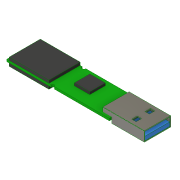
# Autodesk Inventor part: USB stick
Saved by Autodesk Inventor 2017 (Build 210142000, 142)
## iProperties
Part Number: USB stick
Material: Generisch
Document SubType Name: Modeling
Designer: ExCISS
Density: 1 g/cm^3
Appearance: Dunkelgrün
Author: ExCISS
Autodesk Inventor part; units mm, degrees
ref_plane "YZ Plane" through (0, 0, 0) normal (1, 0, 0) x (0, 1, 0)
ref_plane "XZ Plane" through (0, 0, 0) normal (0, 1, 0) x (-1, 0, 0)
ref_plane "XY Plane" through (0, 0, 0) normal (0, 0, 1) x (1, 0, 0)
sketch "Skizze1" plane through (0, 0, 0) normal (0, 0, 1) x (1, 0, 0)
  line L0 (-23.15, 7.05) -> (23.15, 7.05)
  line L1 (23.15, 7.05) -> (23.15, -7.05)
  line L2 (23.15, -7.05) -> (-23.15, -7.05)
  line L3 (-23.15, -7.05) -> (-23.15, 7.05)
  line L4 (-23.15, 7.05) -> (23.15, -7.05) construction
  point P0 (0, 0)
  point P1 (0, 0)
  dimension "d0" = 46.3
  dimension "d1" = 14.1
  constraints: 10 end point, 2 parallel, 1 coincident, 1 horizontal, 1 midpoint, 1 perpendicular
  measures "d0" distance of L1.end L2.end
  measures "d1" distance of L0.end L1.end
extrude "Extrusion1" add sketch "Skizze1" along normal blind 1
sketch "Skizze3" plane through (0, 0, 0) normal (0, 0, 1) x (1, 0, 0)
  line L0 (37.85, 6) -> (19.15, 6)
  line L1 (19.15, 6) -> (19.15, -6)
  line L2 (19.15, -6) -> (37.85, -6)
  line L3 (37.85, -6) -> (37.85, 6)
  line L4 (23.15, -7.05) -> (23.15, 7.05) projected
  line L5 (23.15, 0) -> (19.15, 0) construction
  point P0 (0, 0)
  dimension "d8" = 18.7
  dimension "d9" = 12
  constraints: 10 end point, 2 horizontal, 2 midpoint, 2 parallel, 1 perpendicular
  measures "d8" distance of L2.end L1.end
  measures "d9" distance of L1.end L0.end
extrude "Extrusion2" add sketch "Skizze3" along normal blind 2.9 separate body
sketch "Skizze4" plane through (0, 0, 0) normal (0, 0, -1) x (-1, 0, 0)
  line L0 (-19.15, -6) -> (-37.85, -6) projected
  line L1 (-23.15, -7.05) -> (-23.15, 7.05) projected
  line L2 (-37.85, -6) -> (-23.15, -6)
  line L3 (-23.15, -6) -> (-23.15, 6)
  line L4 (-23.15, 6) -> (-37.85, 6)
  line L5 (-37.85, 6) -> (-37.85, -6)
  point P0 (0, 0)
  dimension "d16" = 12
  constraints: 8 end point, 2 parallel, 1 horizontal, 1 perpendicular, 1 point on line
  measures "d16" distance of L3.end L2.end
extrude "Extrusion3" add sketch "Skizze4" along normal blind 1.6 bodies 2
sketch "Skizze5" plane through (0, 0, 1) normal (0, 0, 1) x (1, 0, 0)
  line L0 (-23.15, 7.05) -> (-23.15, -7.05) construction
  line L1 (23.15, 7.05) -> (-23.15, 7.05) construction
  line L2 (-22.15, 7.05) -> (-4.15, 7.05)
  line L3 (-4.15, 7.05) -> (-4.15, -7.05)
  line L4 (-4.15, -7.05) -> (-22.15, -7.05)
  line L5 (-22.15, -7.05) -> (-22.15, 7.05)
  point P0 (0, 0)
  dimension "d20" = 18
  dimension "d21" = 14.1
  constraints: 8 end point, 2 parallel, 1 horizontal, 1 perpendicular, 1 point on line
  measures "d20" distance of L3.end L4.end
  measures "d21" distance of L2.end L3.end
extrude "Extrusion4" add sketch "Skizze5" along normal blind 1.3 bodies 1
sketch "Skizze6" plane through (0, 0, 0) normal (0, 0, -1) x (-1, 0, 0)
  line L0 (23.15, 7.05) -> (23.15, -7.05) construction
  line L1 (23.15, 0) -> (22.15, 0) construction
  line L2 (22.15, 7.05) -> (22.15, -7.05) projected
  line L3 (22.15, -7.05) -> (4.15, -7.05)
  line L4 (4.15, -7.05) -> (4.15, 7.05)
  line L5 (4.15, 7.05) -> (22.15, 7.05)
  line L6 (22.15, 7.05) -> (22.15, -7.05)
  point P0 (0, 0)
  dimension "d24" = 1
  dimension "d25" = 18
  dimension "d26" = 14.1
  constraints: 10 end point, 2 horizontal, 2 parallel, 1 midpoint, 1 perpendicular
  measures "d24" distance of L1.start L1.end
  measures "d25" distance of L4.end L5.end
  measures "d26" distance of L3.end L4.end
extrude "Extrusion5" add sketch "Skizze6" along normal blind 1.3 bodies 1
sketch "Skizze8" plane through (37.85, -6, 2.9) normal (1, 0, 0) x (0, 0, -1)
  line L0 (4.5, 12) -> (4.5, 0) projected
  line L1 (0, 0) -> (0, 12) projected
  line L2 (0.35, 0.35) -> (2.35, 0.35)
  line L3 (2.35, 0.35) -> (2.35, 11.65)
  line L4 (2.35, 11.65) -> (0.35, 11.65)
  line L5 (0.35, 11.65) -> (0.35, 0.35)
  line L6 (0, 12) -> (0, 0) construction
  line L7 (0, 6) -> (0.35, 6) construction
  dimension "d42" = 2
  dimension "d43" = 11.3
  dimension "d44" = 0.35
  constraints: 10 end point, 2 horizontal, 2 midpoint, 2 parallel, 1 perpendicular
  measures "d42" distance of L4.end L3.end
  measures "d43" distance of L3.end L2.end
  measures "d44" distance of L7.end L7.start
extrude "Extrusion6" cut sketch "Skizze8" against normal blind 9 bodies 2
sketch "Skizze9" plane through (37.85, -6, 2.9) normal (1, 0, 0) x (0, 0, -1)
  line L0 (0, 0) -> (0, 12) projected
  line L1 (4.5, 12) -> (4.5, 0) projected
  line L2 (2.35, 11.65) -> (2.35, 0.35) projected
  line L3 (2.35, 0.35) -> (4.15, 0.35)
  line L4 (4.15, 0.35) -> (4.15, 11.65)
  line L5 (4.15, 11.65) -> (2.35, 11.65)
  line L6 (2.35, 11.65) -> (2.35, 0.35)
  point P0 (2.9, 6)
  constraints: 8 end point, 2 parallel, 1 horizontal, 1 perpendicular
extrude "Extrusion7" cut sketch "Skizze9" against normal blind 0.1 bodies 2
sketch "Skizze15" plane through (0, 0, 1) normal (0, 0, 1) x (1, 0, 0)
  line L0 (-4.1196, -7.0919) -> (-2.4201, -7.05) construction
  line L1 (-4.15, -7.05) -> (23.15, -7.05) construction
  circle A0 centre (-2.4201, -7.05) radius 0.7
  point P0 (0, 0)
  dimension "d81" = 1.7
  dimension "d82" = 1.4
  constraints: 2 end point, 1 centre point, 1 coincident, 1 point on line
  measures "d81" distance of L0.start L0.end
  measures "d82" diameter of A0
extrude "Extrusion8" cut sketch "Skizze15" against normal blind 1 bodies 1
sketch "Skizze17" plane through (0, 0, 1) normal (0, 0, 1) x (1, 0, 0)
  line L0 (-4.15, 7.05) -> (-22.15, 7.05) projected
  line L1 (-4.15, 7.05) -> (-2.45, 7.05)
  line L2 (23.15, 7.05) -> (-4.15, 7.05) projected
  circle A0 centre (-2.45, 7.05) radius 0.85
  point P0 (0, 0)
  dimension "d87" = 1.7
  dimension "d88" = 1.7
  constraints: 2 end point, 1 centre point, 1 coincident, 1 point on line
  measures "d87" distance of L0.start L1.end
  measures "d88" diameter of A0
extrude "Extrusion9" cut sketch "Skizze17" against normal blind 1 bodies 1
sketch "Skizze19" plane through (0, 0, 2.9) normal (0, 0, 1) x (1, 0, 0)
  line L0 (37.85, -6) -> (37.85, 6) projected
  line L1 (32.45, -4.25) -> (30.45, -4.25)
  line L2 (30.45, -4.25) -> (30.45, -1.75)
  line L3 (30.45, -1.75) -> (32.45, -1.75)
  line L4 (32.45, -1.75) -> (32.45, -4.25)
  point P0 (0, 0)
  point P1 (32.45, 4.25)
  dimension "d101" = 2
  dimension "d102" = 2.5
  constraints: 8 end point, 2 parallel, 1 horizontal, 1 perpendicular
  measures "d101" distance of L2.end L3.end
  measures "d102" distance of L1.end L2.end
extrude "Extrusion10" cut sketch "Skizze19" against normal up to next bodies 2
sketch "Skizze20" plane through (0, 0, 2.9) normal (0, 0, 1) x (1, 0, 0)
  line L0 (37.85, 5.65) -> (37.85, -5.65) projected
  line L1 (37.85, 0) -> (32.45, 0)
  line L2 (32.45, 0) -> (32.45, 4.25)
  line L3 (32.45, 4.25) -> (30.45, 4.25)
  line L4 (30.45, 4.25) -> (30.45, 1.75)
  line L5 (30.45, 1.75) -> (32.45, 1.75)
  line L6 (32.45, 1.75) -> (32.45, 4.25)
  point P0 (0, 0)
  dimension "d107" = 5.4
  dimension "d108" = 4.25
  dimension "d109" = 2
  dimension "d110" = 2.5
  constraints: 12 end point, 2 horizontal, 2 parallel, 2 perpendicular, 1 midpoint
  measures "d107" distance of L1.start L1.end
  measures "d108" distance of L1.end L2.end
  measures "d109" distance of L5.end L4.end
  measures "d110" distance of L4.end L3.end
extrude "Extrusion11" cut sketch "Skizze20" against normal up to next bodies 2
fillet "Rundung1" radius 0.1 2 edges at (28.5, -6, 2.9) (28.5, 6, 2.9)
fillet "Rundung3" radius 0.1 1 edges at (30.5, -6, -1.6)
fillet "Rundung4" radius 0.1 1 edges at (30.5, 6, -1.6)
fillet "Rundung5" radius 0.1 1 edges at (37.8, -5.65, -1.25)
fillet "Rundung6" radius 0.1 1 edges at (33.35, -5.65, 2.55)
fillet "Rundung7" radius 0.1 1 edges at (37.8, 5.65, -1.25)
fillet "Rundung8" radius 0.1 1 edges at (33.35, 5.65, 2.55)
sketch "Skizze21" plane through (0, 0, 1) normal (0, 0, 1) x (1, 0, 0)
  line L0 (2.45, 4.81) -> (9.49, 4.81)
  line L1 (9.49, 4.81) -> (9.49, -2.23)
  line L2 (9.49, -2.23) -> (2.45, -2.23)
  line L3 (2.45, -2.23) -> (2.45, 4.81)
  line L4 (19.15, 5.9) -> (19.15, -5.9) construction
  line L5 (-4.15, -7.05) -> (-4.15, 7.05) construction
  line L6 (-4.15, 7.05) -> (2.45, 7.05) construction
  line L7 (2.45, 7.05) -> (2.45, 4.81) construction
  line L8 (2.45, 4.81) -> (-4.15, 4.81) construction
  line L9 (-4.15, 4.81) -> (-4.15, 7.05) construction
  point P0 (0, 0)
  dimension "d121" = 7.04
  dimension "d122" = 7.04
  dimension "d125" = 6.6
  dimension "d126" = 2.24
  constraints: 16 end point, 4 parallel, 2 horizontal, 2 perpendicular
  measures "d121" distance of L1.end L2.end
  measures "d122" distance of L0.end L1.end
  measures "d125" distance of L0.start L8.end
  measures "d126" distance of L6.end L0.start
extrude "Extrusion12" add sketch "Skizze21" along normal blind 1.1 bodies 1
sketch "Skizze22" plane through (-23.15, -7.05, 0) normal (0, -1, 0) x (1, 0, 0)
  line L0 (19, 2.3) -> (1, 2.3) projected
  line L1 (19, 1) -> (20.0299, 1) projected
  line L2 (1, 2.3) -> (19, 2.3)
  line L3 (19, 2.3) -> (19, 1)
  line L4 (19, 1) -> (1, 1)
  line L5 (1, 1) -> (1, 2.3)
  line L6 (1, -1.3) -> (19, -1.3) projected
  line L7 (19, 0) -> (1, 0)
  line L8 (1, 0) -> (1, -1.3)
  line L9 (1, -1.3) -> (19, -1.3)
  line L10 (19, -1.3) -> (19, 0)
  point P0 (23.15, 0)
  constraints: 16 end point, 4 parallel, 2 horizontal, 2 perpendicular
extrude "Extrusion13" cut sketch "Skizze22" against normal blind 0.001 bodies 1
sketch "Skizze23" plane through (-23.15, 7.05, 1) normal (0, 1, 0) x (1, 0, 0)
  line L0 (19, 0) -> (19, -1.3) projected
  line L1 (19, -1.3) -> (1, -1.3)
  line L2 (1, -1.3) -> (1, 0)
  line L3 (1, 0) -> (19, 0)
  line L4 (19, 0) -> (19, -1.3)
  line L5 (1, 1) -> (1, 2.3) projected
  line L6 (19, 1) -> (19, 2.3) projected
  line L7 (1, 1) -> (19, 1)
  line L8 (19, 1) -> (19, 2.3)
  line L9 (19, 2.3) -> (1, 2.3)
  line L10 (1, 2.3) -> (1, 1)
  point P0 (23.15, 1)
  constraints: 16 end point, 4 parallel, 2 horizontal, 2 perpendicular
extrude "Extrusion14" add sketch "Skizze23" along normal blind 0.001 bodies 1
